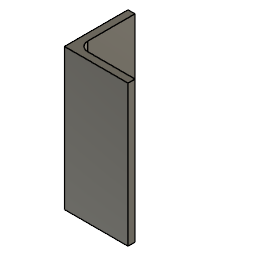
L-45×45×5 (Autodesk Fusion 360 design; units mm, degrees)
Autodesk Fusion 360 part; units mm, degrees
sketch "スケッチ1" plane through (0, 0, 0) normal (0, 0, 1) x (1, 0, 0)
  arc A0 (5, 11.5) -> (11.5, 5) centre (11.5, 11.5) ccw
  line L0 (0, 45) -> (0, 0)
  line L1 (45, 5) -> (11.5, 5)
  line L2 (0, 0) -> (45, 0)
  line L3 (45, 0) -> (45, 5)
  line L4 (5, 11.5) -> (5, 45)
  line L5 (5, 45) -> (0, 45)
extrude "押し出し1" add sketch "スケッチ1" along normal blind 100
